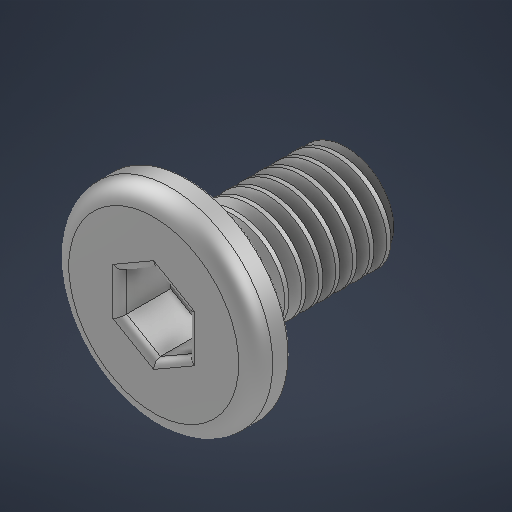
# Autodesk Inventor part: M3 x5L_hexagonal
Saved by Autodesk Inventor 2025.2 (Build 292293000, 293)
## iProperties
Created: 2024-12-01
Part Number: M3 x5L_hexagonal
Material: Generic
Document SubType Name: Modeling
Designer: Tiago
Density: 1 g/cm^3
Appearance: Anodized - Light Gray
Author: Tiago
Autodesk Inventor part; units mm, degrees
ref_plane "YZ Plane" through (0, 0, 0) normal (1, 0, 0) x (0, 1, 0)
ref_plane "XZ Plane" through (0, 0, 0) normal (0, 1, 0) x (-1, 0, 0)
sketch "Sketch2" plane through (0, 0, 0) normal (0, 1, 0) x (-1, 0, 0)
  line L0 (0, 0) -> (0, -6)
  line L1 (-0.8865, -6) -> (-0.8865, -1)
  line L2 (-3, 0) -> (-3, -1)
  line L3 (-3, -1) -> (-0.8865, -1)
  line L4 (-0.8865, -6) -> (0, -6)
  line L5 (0, -6) -> (-1.5, -6)
  line L6 (-1.5, -6) -> (-1.5, -8.4311)
  line L7 (-1.5, -8.4311) -> (0, -8.4311)
  line L8 (0, -8.4311) -> (0, -6)
  line L9 (-1.5, -6) -> (-1.5, -5.4)
  line L10 (-0.8865, -6) -> (-1.5, -5.6458)
  line L11 (-3, 0) -> (0, 0)
  dimension "d0" = 1.773
  dimension "d79" = 6
  dimension "d84" = 3
  dimension "d91" = 30
  dimension "x" = 1
  dimension "d94" = 2.4311
  dimension "d98" = 0.6
  dimension "d103" = 5
  constraints: 25 end point, 3 horizontal, 3 parallel, 3 vertical, 2 horizontal alignment, 2 perpendicular, 1 point on line
  measures "d0" diameter of L1 L0
  measures "d79" diameter of L2.start L0
  measures "d84" diameter of L6 L0
  measures "d91" angle of L5 L10
  measures "x" distance from line of L0.start L3
  measures "d94" distance between parallel lines of L4 L7
  measures "d98" distance from line of L5 L9.end
  measures "d103" distance between parallel lines of L4 L3
revolve "Revolution1" add sketch "Sketch2" angle 360 about axis through (0, 0, 0) along (0, 0, -1) contours L0 L4 L1 L3 L2 L11
sketch "Sketch4" plane through (0, 0, 0) normal (0, 1, 0) x (-1, 0, 0)
  line L0 (0, -13.6001) -> (0, 2.2667) projected
  line L1 (-1.5, -6.8542) -> (-1.5, -6.9792)
  line L2 (-1.5, -6.9792) -> (-0.8865, -7.3334)
  line L3 (-0.8865, -7.3334) -> (-0.8865, -6.5)
  line L4 (-1.5, -6.8542) -> (-0.8865, -6.5)
  line L5 (-1.5, -6.9167) -> (-0.8865, -6.9167)
  line L6 (0, -10) -> (0, -9)
  line L7 (2.1429, -9) -> (-2.1429, -9)
  line L8 (-0.8865, -1) -> (-3, -1) projected
  line L9 (-3, -1) -> (-3, 0) projected
  line L10 (3, 0) -> (3, -1) projected
  line L11 (3, -1) -> (0.8865, -1) projected
  line L12 (0.8865, -1) -> (0.8865, -6) projected
  line L13 (-0.8865, -6) -> (-0.8865, -1) projected
  line L14 (0.8865, -6) -> (-0.8865, -6) projected
  line L15 (-3, 0) -> (3, 0) projected
  point P0 (0, 0)
  point P1 (-1.5, -6.3542)
  point P2 (0, -10.9667)
  dimension "d" = 1.773
  dimension "d28" = 0.5
  dimension "d77" = 0.125
  dimension "d78" = 60
  dimension "d81" = 0.5
  dimension "d90" = 0.6135
  constraints: 14 end point, 3 midpoint, 3 point on line, 2 horizontal, 1 equal length, 1 parallel, 1 vertical
  measures "d" diameter of L3 L0
  measures "d28" distance of point (-1.5, -6.354) L1.start
  measures "d77" distance of L1.start L1.end
  measures "d78" angle of L2 L4
  measures "d81" distance of L13.start L3.end
  measures "d90" distance of L5.start L5.end
coil "Coil1" sketch "Sketch4" operation add axis through (0, 0, -10) along (0, 0, 1) pitch 0.5 turns 12.3 hand right contours L4 L3 L5 L1 | L5 L3 L2 L1
ref_plane "Work Plane1" through (0, 0, -3) normal (0, 0, 1) x (1, 0, 0)
revolve "Revolution3" cut sketch "Sketch2" angle 360 about axis through (0, 0, 0) along (0, 0, -1) contours L8 L7 L6 L5 L4 | L5 L9 L10
fillet "Fillet4" radius 0.5 1 edges at (-3, 0, 0)
sketch "Sketch7" plane through (0, 0, 0) normal (0, 0, 1) x (1, 0, 0)
  line L0 (0, -1.1547) -> (-1, -0.5774)
  line L1 (-1, -0.5774) -> (-1, 0.5774)
  line L2 (-1, 0.5774) -> (0, 1.1547)
  line L3 (0, 1.1547) -> (1, 0.5774)
  line L4 (1, 0.5774) -> (1, -0.5774)
  line L5 (1, -0.5774) -> (0, -1.1547)
  point P0 (0, 0)
  point P1 (0, 0)
  point P2 (1, 0)
  dimension "d99" = 2
  constraints: 12 end point, 1 coincident, 1 horizontal alignment, 1 midpoint, 13 other
  measures "d99" distance between parallel lines of L1 L4
extrude "Extrusion5" cut sketch "Sketch7" against normal blind 1.5
fillet "Fillet5" radius 0.2 6 edges at (0.5, 0.866, 0) (1, 0, 0) (0.5, -0.866, 0) (-0.5, -0.866, 0) (-1, 0, 0) (-0.5, 0.866, 0)
fillet "Fillet6" radius 0.05 1 edges at (-3, 0, -1)
equation "\"M\" = 3"
body "Solid1"
